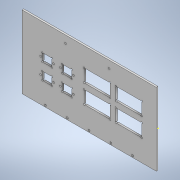
# Autodesk Inventor part: sheetmetalface2.0
Saved by Autodesk Inventor 2020.2 (Build 242310000, 310)
## iProperties
Created: 2020-02-06
Part Number: sheetmetalface2.0
Material: Generic
Document SubType Name: Sheet Metal
Designer: ColinP
Density: 1 g/cm^3
Sheet Metal Rule: Default
Appearance: Default
Mass: 74.7807 g
Surface Area: 544.759 cm^2
Volume: 74.7807 cm^3
Author: ColinP
Autodesk Inventor part; units mm, degrees
ref_plane "YZ Plane" through (0, 0, 0) normal (1, 0, 0) x (0, 1, 0)
ref_plane "XZ Plane" through (0, 0, 0) normal (0, 1, 0) x (-1, 0, 0)
ref_plane "XY Plane" through (0, 0, 0) normal (0, 0, 1) x (1, 0, 0)
sketch "Sketch1" plane through (0, 0, 0) normal (0, 0, 1) x (1, 0, 0)
  line L0 (120.396, 63.5) -> (-114.3, 63.5)
  line L1 (-114.3, 63.5) -> (-114.3, -63.5)
  line L2 (-114.3, -63.5) -> (120.396, -63.5)
  line L3 (120.396, -63.5) -> (120.396, 63.5)
  point P0 (0, 0)
  dimension "d0" = 234.696
  dimension "d1" = 127
  measures "d0" distance of L2.end L1.end
  measures "d1" distance of L1.end L0.end
extrude "Plate1" add sketch "Sketch1" along normal blind 3.048
sketch "Sketch2" plane through (0, 0, 3.048) normal (0, 0, 1) x (1, 0, 0)
  line L0 (-114.3, 63.5) -> (-114.3, -63.5) projected
  line L1 (-114.3, -63.5) -> (-114.3, -60.325)
  line L2 (-114.3, -60.325) -> (-73.152, -60.325)
  line L3 (-73.152, -60.325) -> (-35.052, -60.325)
  line L4 (-35.052, -60.325) -> (3.048, -60.325)
  line L5 (3.048, -60.325) -> (41.148, -60.325)
  line L6 (41.148, -60.325) -> (79.248, -60.325)
  line L7 (79.248, -60.325) -> (120.396, -60.325)
  line L8 (120.396, -63.5) -> (120.396, 63.5) projected
  point P0 (0, 0)
  dimension "d3" = 3.175
  dimension "d4" = 41.148
  dimension "d5" = 38.1
  dimension "d6" = 38.1
  dimension "d7" = 180
  dimension "d8" = 38.1
  dimension "d9" = 38.1
  constraints: 14 end point, 5 point on line, 1 collinear, 1 horizontal, 1 perpendicular
  measures "d3" distance of L0.end L1.end
  measures "d4" distance of L1.end L2.end
  measures "d5" distance of L2.end L3.end
  measures "d6" distance of L3.end L4.end
  measures "d7" angle of L4 L3
  measures "d8" distance of L4.end L5.end
  measures "d9" distance of L5.end L6.end
hole "Hole1" at (-73.152, -60.325, 3.048) at (-35.052, -60.325, 3.048) at (3.048, -60.325, 3.048) at (41.148, -60.325, 3.048) at (79.248, -60.325, 3.048) direction (0, 0, -1) diameter 3.2766 depth 8.8646 clearance for "Hex Machine Screw" size "#4" standard "Ansi Unified Screw Threads"
sketch "Sketch3" plane through (0, 0, 3.048) normal (0, 0, 1) x (1, 0, 0)
  line L0 (120.396, -63.5) -> (120.396, 63.5) projected
  line L1 (120.396, -63.5) -> (120.396, -50.8)
  line L2 (120.396, -50.8) -> (120.396, -25.4)
  line L3 (120.396, -25.4) -> (94.996, -25.4)
  line L4 (94.996, -25.4) -> (94.996, -2.794)
  line L5 (94.996, -2.794) -> (49.784, -2.794)
  line L6 (49.784, -2.794) -> (49.784, -25.4)
  line L7 (49.784, -25.4) -> (94.996, -25.4)
  line L8 (94.996, -2.794) -> (94.996, 7.366)
  line L9 (94.996, 7.366) -> (49.784, 7.366)
  line L10 (49.784, 7.366) -> (49.784, 29.972)
  line L11 (49.784, 29.972) -> (94.996, 29.972)
  line L12 (94.996, 29.972) -> (94.996, 7.366)
  line L13 (49.784, 29.972) -> (39.624, 29.972)
  line L14 (39.624, 29.972) -> (39.624, 7.366)
  line L15 (39.624, 7.366) -> (-5.588, 7.366)
  line L16 (-5.588, 7.366) -> (-5.588, 29.972)
  line L17 (-5.588, 29.972) -> (39.624, 29.972)
  line L18 (49.784, -2.794) -> (39.624, -2.794)
  line L19 (39.624, -2.794) -> (39.624, -25.4)
  line L20 (39.624, -25.4) -> (-5.588, -25.4)
  line L21 (-5.588, -25.4) -> (-5.588, -2.794)
  line L22 (-5.588, -2.794) -> (39.624, -2.794)
  point P0 (0, 0)
  dimension "d17" = 12.7
  dimension "d18" = 25.4
  dimension "d19" = 25.4
  dimension "d20" = 22.606
  dimension "d21" = 45.212
  dimension "d22" = 90
  dimension "d23" = 10.16
  dimension "d24" = 22.606
  dimension "d25" = 10.16
  dimension "d26" = 45.212
  constraints: 44 end point, 14 perpendicular, 11 point on line, 1 horizontal, 1 vertical
  measures "d17" distance of L0.start L1.end
  measures "d18" distance of L1.end L2.end
  measures "d19" distance of L2.end L3.end
  measures "d20" distance of L3.end L4.end
  measures "d21" distance of L4.end L5.end
  measures "d22" angle of L5 L4
  measures "d23" distance of L4.end L8.end
  measures "d24" distance of L9.end L10.end
  measures "d25" distance of L10.end L13.end
  measures "d26" distance of L14.end L15.end
extrude "Cut1" cut sketch "Sketch3" against normal blind 3.048
sketch "Sketch4" plane through (0, 0, 3.048) normal (0, 0, 1) x (1, 0, 0)
  line L0 (-114.3, 63.5) -> (-114.3, -63.5) projected
  line L1 (-114.3, -63.5) -> (-114.3, -50.8)
  line L2 (-114.3, -50.8) -> (-78.74, -50.8)
  line L3 (-78.74, -50.8) -> (-78.74, -25.4)
  line L4 (-78.74, -25.4) -> (-61.976, -25.4)
  line L5 (-61.976, -25.4) -> (-61.976, -11.43)
  line L6 (-61.976, -11.43) -> (-78.74, -11.43)
  line L7 (-78.74, -11.43) -> (-78.74, -25.4)
  line L8 (-61.976, -11.43) -> (-44.196, -11.43)
  line L9 (-44.196, -11.43) -> (-27.432, -11.43)
  line L10 (-27.432, -11.43) -> (-27.432, -25.4)
  line L11 (-27.432, -25.4) -> (-44.196, -25.4)
  line L12 (-44.196, -25.4) -> (-44.196, -11.43)
  line L13 (-44.196, -11.43) -> (-44.196, 2.54)
  line L14 (-44.196, 2.54) -> (-44.196, 16.51)
  line L15 (-44.196, 16.51) -> (-27.432, 16.51)
  line L16 (-27.432, 16.51) -> (-27.432, 2.54)
  line L17 (-27.432, 2.54) -> (-44.196, 2.54)
  line L18 (-44.196, 2.54) -> (-61.976, 2.54)
  line L19 (-61.976, 16.51) -> (-61.976, 2.54)
  line L20 (-61.976, 2.54) -> (-78.74, 2.54)
  line L21 (-78.74, 16.51) -> (-61.976, 16.51)
  line L22 (-78.74, 16.51) -> (-78.74, 2.54)
  point P0 (0, 0)
  dimension "d29" = 12.7
  dimension "d30" = 35.56
  dimension "d31" = 25.4
  dimension "d32" = 16.764
  dimension "d33" = 13.97
  dimension "d34" = 17.78
  dimension "d35" = 16.764
  dimension "d36" = 13.97
  dimension "d37" = 13.97
  constraints: 44 end point, 17 point on line, 11 perpendicular, 1 horizontal, 1 parallel
  measures "d29" distance of L0.end L1.end
  measures "d30" distance of L1.end L2.end
  measures "d31" distance of L2.end L3.end
  measures "d32" distance of L3.end L4.end
  measures "d33" distance of L4.end L5.end
  measures "d34" distance of L5.end L8.end
  measures "d35" distance of L8.end L9.end
  measures "d36" distance of L8.end L13.end
  measures "d37" distance of L13.end L14.end
extrude "Cut2" cut sketch "Sketch4" against normal blind 3.048
sketch "Sketch5" plane through (120.396, -63.5, 0) normal (1, 0, 0) x (0, 0, -1)
  point P0 (0, 63.5)
sketch "Sketch6" plane through (0, 0, 3.048) normal (0, 0, 1) x (1, 0, 0)
  line L0 (120.396, 63.5) -> (-114.3, 63.5) projected
  line L1 (-114.3, 63.5) -> (-114.3, 50.8)
  line L2 (-114.3, 63.5) -> (-114.3, -63.5) projected
  line L3 (-114.3, 50.8) -> (-38.1, 50.8)
  line L4 (-38.1, 50.8) -> (38.1, 50.8)
  point P0 (0, 0)
  dimension "d40" = 12.7
  dimension "d41" = 76.2
  dimension "d42" = 270
  dimension "d43" = 76.2
  constraints: 6 end point, 2 point on line, 1 perpendicular
  measures "d40" distance of L0.end L1.end
  measures "d41" distance of L1.end L3.end
  measures "d43" distance of L3.end L4.end
hole "Hole2" at (-38.1, 50.8, 3.048) at (38.1, 50.8, 3.048) direction (0, 0, -1) diameter 3.2766 end through all clearance for "Flat Head Machine Screw (82)" size "#4" standard "Ansi Unified Screw Threads"
sketch "Sketch7" plane through (0, 0, 3.048) normal (0, 0, 1) x (1, 0, 0)
  line L0 (-61.976, 2.54) -> (-61.976, 16.51) projected
  line L1 (-61.976, 9.525) -> (-58.928, 9.525)
  line L2 (-58.928, 9.525) -> (-52.324, 9.525)
  line L3 (-52.324, 9.525) -> (-52.324, -18.415)
  line L4 (-44.196, -11.43) -> (-44.196, -25.4) projected
  line L5 (-52.324, -18.415) -> (-78.74, -18.415)
  line L6 (-78.74, -11.43) -> (-78.74, -25.4) projected
  line L7 (-78.74, -18.415) -> (-81.7878, -18.3763)
  line L8 (-81.7878, -18.3763) -> (-81.4331, 9.525)
  line L9 (-81.4331, 9.525) -> (-27.432, 9.525)
  line L10 (-27.432, 2.54) -> (-27.432, 16.51) projected
  line L11 (-27.432, 9.525) -> (-24.384, 9.525)
  line L12 (-24.384, 9.525) -> (-24.384, -19.1059)
  line L13 (-52.324, 9.525) -> (-38.3228, 9.525)
  line L14 (-38.3228, 9.525) -> (-41.3708, 9.525)
  line L15 (-41.3708, 9.525) -> (-41.3708, -18.415)
  line L16 (-61.976, -25.4) -> (-61.976, -11.43) projected
  line L17 (-61.976, -18.415) -> (-58.928, -18.415)
  line L18 (-44.196, 2.54) -> (-44.196, 16.51) projected
  line L19 (-38.3228, 9.525) -> (-41.3708, 9.525)
  line L20 (-44.196, 9.525) -> (-47.244, 9.525)
  line L21 (-47.244, 9.525) -> (-47.244, -18.415)
  point P0 (0, 0)
  dimension "d51" = 3.048
  dimension "d52" = 6.604
  dimension "d53" = 3.048
  dimension "d54" = 3.048
  dimension "d62" = 3.048
  dimension "d63" = 3.048
  dimension "d78" = 3.048
  constraints: 32 end point, 8 point on line, 5 midpoint, 5 perpendicular, 2 horizontal, 1 parallel, 4 other
  measures "d51" distance of L1.start L1.end
  measures "d52" distance of L1.end L2.end
  measures "d53" distance of L7.start L7.end
  measures "d54" distance of L9.end L11.end
  measures "d62" distance of L13.end L14.end
  measures "d63" distance of L17.start L17.end
  measures "d78" distance of L20.start L20.end
hole "Hole3" at (-81.4331, 9.525, 3.048) at (-81.7878, -18.3763, 3.048) at (-24.384, -19.1059, 3.048) at (-24.384, 9.525, 3.048) at (-58.928, 9.525, 3.048) at (-58.928, -18.415, 3.048) at (-41.3708, -18.415, 3.048) at (-41.3708, 9.525, 3.048) at (-47.244, 9.525, 3.048) at (-47.244, -18.415, 3.048) direction (0, 0, -1) diameter 3.048 depth 3.048
sketch "Sketch8" plane through (0, 0, 3.048) normal (0, 0, 1) x (1, 0, 0)
  circle A0 centre (-58.928, 9.525) radius 1.524 projected
  circle A1 centre (-24.384, -19.1059) radius 1.524 projected
  circle A2 centre (-81.4331, 9.525) radius 1.524 projected
  circle A3 centre (-81.7878, -18.3763) radius 1.524 projected
  circle A4 centre (-24.384, 9.525) radius 1.524 projected
  circle A5 centre (-58.928, -18.415) radius 1.524 projected
  circle A6 centre (-38.1, 50.8) radius 1.6383 projected
  circle A7 centre (38.1, 50.8) radius 1.6383 projected
  line L0 (-27.432, -25.4) -> (-44.196, -25.4) projected
  line L1 (-44.196, -25.4) -> (-44.196, -11.43) projected
  line L2 (-44.196, -11.43) -> (-27.432, -11.43) projected
  line L3 (-27.432, -11.43) -> (-27.432, -25.4) projected
  line L4 (-78.74, 16.51) -> (-61.976, 16.51) projected
  line L5 (-61.976, 16.51) -> (-61.976, 2.54) projected
  line L6 (-61.976, 2.54) -> (-78.74, 2.54) projected
  line L7 (-78.74, 2.54) -> (-78.74, 16.51) projected
  line L8 (-27.432, 16.51) -> (-27.432, 2.54) projected
  line L9 (-27.432, 2.54) -> (-44.196, 2.54) projected
  line L10 (-44.196, 2.54) -> (-44.196, 16.51) projected
  line L11 (-44.196, 16.51) -> (-27.432, 16.51) projected
  line L12 (-61.976, -11.43) -> (-61.976, -25.4) projected
  line L13 (-61.976, -25.4) -> (-78.74, -25.4) projected
  line L14 (-78.74, -25.4) -> (-78.74, -11.43) projected
  line L15 (-78.74, -11.43) -> (-61.976, -11.43) projected
  line L16 (49.784, 29.972) -> (94.996, 29.972) projected
  line L17 (94.996, 29.972) -> (94.996, 7.366) projected
  line L18 (94.996, 7.366) -> (49.784, 7.366) projected
  line L19 (49.784, 7.366) -> (49.784, 29.972) projected
  line L20 (-5.588, -25.4) -> (-5.588, -2.794) projected
  line L21 (-5.588, -2.794) -> (39.624, -2.794) projected
  line L22 (39.624, -2.794) -> (39.624, -25.4) projected
  line L23 (39.624, -25.4) -> (-5.588, -25.4) projected
  line L24 (-5.588, 7.366) -> (-5.588, 29.972) projected
  line L25 (-5.588, 29.972) -> (39.624, 29.972) projected
  line L26 (39.624, 29.972) -> (39.624, 7.366) projected
  line L27 (39.624, 7.366) -> (-5.588, 7.366) projected
  line L28 (49.784, -2.794) -> (94.996, -2.794) projected
  line L29 (94.996, -2.794) -> (94.996, -25.4) projected
  line L30 (94.996, -25.4) -> (49.784, -25.4) projected
  line L31 (49.784, -25.4) -> (49.784, -2.794) projected
  circle A8 centre (41.148, -60.325) radius 1.6383 projected
  circle A9 centre (-35.052, -60.325) radius 1.6383 projected
  circle A10 centre (-73.152, -60.325) radius 1.6383 projected
  circle A11 centre (3.048, -60.325) radius 1.6383 projected
  circle A12 centre (79.248, -60.325) radius 1.6383 projected
  line L32 (120.396, 63.5) -> (120.396, -63.5) projected
  line L33 (-114.3, 63.5) -> (120.396, 63.5) projected
  line L34 (-114.3, -63.5) -> (-114.3, 63.5) projected
  line L35 (120.396, -63.5) -> (-114.3, -63.5) projected
  point P0 (0, 0)
  point P1 (-119.4297, -23.9926)
hole "Hole4" at (-78.74, 16.51, 3.048) at (-61.976, 16.51, 3.048) at (-61.976, 2.54, 3.048) at (-78.74, 2.54, 3.048) at (-78.74, -11.43, 3.048) at (-61.976, -11.43, 3.048) at (-61.976, -25.4, 3.048) at (-78.74, -25.4, 3.048) at (-44.196, -25.4, 3.048) at (-27.432, -25.4, 3.048) at (-27.432, -11.43, 3.048) at (-119.4297, -23.9926, 3.048) at (-44.196, -11.43, 3.048) at (-44.196, 2.54, 3.048) at (-44.196, 16.51, 3.048) at (-27.432, 16.51, 3.048) at (-27.432, 2.54, 3.048) direction (0, 0, -1) diameter 2.4384 depth 3.048 clearance for "Flat Head Machine Screw (82)" size "#2" standard "Ansi Unified Screw Threads"
sketch "Sketch9" plane through (0, 0, 3.048) normal (0, 0, 1) x (1, 0, 0)
  arc A0 (-27.432, 15.2908) -> (-28.6512, 16.51) centre (-27.432, 16.51) ccw projected
  line L0 (-27.432, 15.2908) -> (-27.432, 3.7592) projected
  arc A1 (-28.6512, 2.54) -> (-27.432, 3.7592) centre (-27.432, 2.54) ccw projected
  line L1 (-28.6512, 2.54) -> (-42.9768, 2.54) projected
  arc A2 (-44.196, 3.7592) -> (-42.9768, 2.54) centre (-44.196, 2.54) ccw projected
  line L2 (-44.196, 3.7592) -> (-44.196, 15.2908) projected
  arc A3 (-42.9768, 16.51) -> (-44.196, 15.2908) centre (-44.196, 16.51) ccw projected
  line L3 (-42.9768, 16.51) -> (-28.6512, 16.51) projected
  arc A4 (-28.6512, -25.4) -> (-27.432, -24.1808) centre (-27.432, -25.4) ccw projected
  line L4 (-28.6512, -25.4) -> (-42.9768, -25.4) projected
  arc A5 (-44.196, -24.1808) -> (-42.9768, -25.4) centre (-44.196, -25.4) ccw projected
  line L5 (-44.196, -24.1808) -> (-44.196, -12.6492) projected
  arc A6 (-42.9768, -11.43) -> (-44.196, -12.6492) centre (-44.196, -11.43) ccw projected
  line L6 (-42.9768, -11.43) -> (-28.6512, -11.43) projected
  arc A7 (-27.432, -12.6492) -> (-28.6512, -11.43) centre (-27.432, -11.43) ccw projected
  line L7 (-27.432, -12.6492) -> (-27.432, -24.1808) projected
  arc A8 (-78.74, -24.1808) -> (-77.5208, -25.4) centre (-78.74, -25.4) ccw projected
  line L8 (-78.74, -24.1808) -> (-78.74, -12.6492) projected
  arc A9 (-77.5208, -11.43) -> (-78.74, -12.6492) centre (-78.74, -11.43) ccw projected
  line L9 (-77.5208, -11.43) -> (-63.1952, -11.43) projected
  arc A10 (-61.976, -12.6492) -> (-63.1952, -11.43) centre (-61.976, -11.43) ccw projected
  line L10 (-61.976, -12.6492) -> (-61.976, -24.1808) projected
  arc A11 (-63.1952, -25.4) -> (-61.976, -24.1808) centre (-61.976, -25.4) ccw projected
  line L11 (-63.1952, -25.4) -> (-77.5208, -25.4) projected
  arc A12 (-78.74, 3.7592) -> (-77.5208, 2.54) centre (-78.74, 2.54) ccw projected
  line L12 (-78.74, 3.7592) -> (-78.74, 15.2908) projected
  arc A13 (-77.5208, 16.51) -> (-78.74, 15.2908) centre (-78.74, 16.51) ccw projected
  line L13 (-77.5208, 16.51) -> (-63.1952, 16.51) projected
  arc A14 (-61.976, 15.2908) -> (-63.1952, 16.51) centre (-61.976, 16.51) ccw projected
  line L14 (-61.976, 15.2908) -> (-61.976, 3.7592) projected
  arc A15 (-63.1952, 2.54) -> (-61.976, 3.7592) centre (-61.976, 2.54) ccw projected
  line L15 (-63.1952, 2.54) -> (-77.5208, 2.54) projected
  circle A16 centre (-58.928, 9.525) radius 1.524 projected
  circle A17 centre (-24.384, -19.1059) radius 1.524 projected
  circle A18 centre (-81.4331, 9.525) radius 1.524 projected
  circle A19 centre (-81.7878, -18.3763) radius 1.524 projected
  circle A20 centre (-24.384, 9.525) radius 1.524 projected
  circle A21 centre (-58.928, -18.415) radius 1.524 projected
  circle A22 centre (-38.1, 50.8) radius 1.6383 projected
  circle A23 centre (38.1, 50.8) radius 1.6383 projected
  line L16 (49.784, 29.972) -> (94.996, 29.972) projected
  line L17 (94.996, 29.972) -> (94.996, 7.366) projected
  line L18 (94.996, 7.366) -> (49.784, 7.366) projected
  line L19 (49.784, 7.366) -> (49.784, 29.972) projected
  line L20 (-5.588, -25.4) -> (-5.588, -2.794) projected
  line L21 (-5.588, -2.794) -> (39.624, -2.794) projected
  line L22 (39.624, -2.794) -> (39.624, -25.4) projected
  line L23 (39.624, -25.4) -> (-5.588, -25.4) projected
  line L24 (-5.588, 7.366) -> (-5.588, 29.972) projected
  line L25 (-5.588, 29.972) -> (39.624, 29.972) projected
  line L26 (39.624, 29.972) -> (39.624, 7.366) projected
  line L27 (39.624, 7.366) -> (-5.588, 7.366) projected
  line L28 (49.784, -2.794) -> (94.996, -2.794) projected
  line L29 (94.996, -2.794) -> (94.996, -25.4) projected
  line L30 (94.996, -25.4) -> (49.784, -25.4) projected
  line L31 (49.784, -25.4) -> (49.784, -2.794) projected
  circle A24 centre (41.148, -60.325) radius 1.6383 projected
  circle A25 centre (-35.052, -60.325) radius 1.6383 projected
  circle A26 centre (-73.152, -60.325) radius 1.6383 projected
  circle A27 centre (3.048, -60.325) radius 1.6383 projected
  circle A28 centre (79.248, -60.325) radius 1.6383 projected
  line L32 (120.396, 63.5) -> (120.396, -63.5) projected
  line L33 (-114.3, 63.5) -> (120.396, 63.5) projected
  line L34 (-114.3, -63.5) -> (-114.3, 63.5) projected
  line L35 (120.396, -63.5) -> (-114.3, -63.5) projected
  point P0 (0, 0)
  point P1 (24.9581, 18.3888)
hole "Hole5" at (-5.588, 29.972, 3.048) at (-5.588, 7.366, 3.048) at (39.624, 7.366, 3.048) at (39.624, 29.972, 3.048) at (24.9581, 18.3888, 3.048) at (49.784, 29.972, 3.048) at (49.784, 7.366, 3.048) at (94.996, 7.366, 3.048) at (94.996, 29.972, 3.048) at (94.996, -2.794, 3.048) at (94.996, -25.4, 3.048) at (49.784, -25.4, 3.048) at (49.784, -2.794, 3.048) at (-5.588, -2.794, 3.048) at (-5.588, -25.4, 3.048) at (39.624, -25.4, 3.048) at (39.624, -2.794, 3.048) direction (0, 0, -1) diameter 2.794 depth 3.048 clearance for "Flat Head Machine Screw (82)" size "#3" standard "Ansi Unified Screw Threads"
equation "\"d27\" = Thickness"
equation "\"d38\" = Thickness"
equation "\"d49\" = Thickness"
equation "\"d60\" = Thickness"
equation "\"d69\" = Thickness"
equation "\"d76\" = Thickness"
equation "\"d2\" = Thickness"
equation "\"BendRadius\" = Thickness"
equation "\"BendReliefWidth\" = Thickness"
equation "\"BendReliefDepth\" = 0.5 * Thickness"
equation "\"CornerReliefSize\" = 4 * Thickness"
equation "\"MinimumRemnant\" = 2 * Thickness"
equation "\"TransitionRadius\" = BendRadius"
equation "\"JacobiRadiusSize\" = BendRadius"
equation "\"GapSize\" = Thickness"
equation "\"Thickness\" = 3.048"
body "Solid1"
